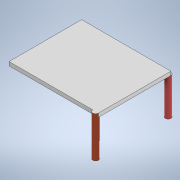
# Autodesk Inventor part: 零件3
Saved by Autodesk Inventor 2022 (Build 260153000, 153)
## iProperties
Created: 2023-03-09
Part Number: 零件3
Material: 一般
Document SubType Name: Modeling
Designer: JOU
Density: 1 g/cm^3
Appearance: 預設
Author: JOU
Autodesk Inventor part; units mm, degrees
ref_plane "YZ Plane" through (0, 0, 0) normal (1, 0, 0) x (0, 1, 0)
ref_plane "XZ Plane" through (0, 0, 0) normal (0, 1, 0) x (-1, 0, 0)
ref_plane "XY Plane" through (0, 0, 0) normal (0, 0, 1) x (1, 0, 0)
sketch "草圖1" plane through (0, 0, 0) normal (0, 1, 0) x (-1, 0, 0)
  circle A0 centre (0.913, -0.7631) radius 0.75
  point P0 (0, 0)
  dimension "d0" = 1.5
  constraints: 1 centre point
  measures "d0" diameter of A0
extrude "擠出1" add sketch "草圖1" along normal blind 10
sketch "草圖2" plane through (-0.913, 10, -0.7631) normal (0, 1, 0) x (1, 0, 0)
  circle A0 centre (0, 0) radius 0.75 projected
  line L0 (-0.75, 0) -> (0.75, 0)
  line L1 (0.75, 0) -> (0.75, 19.5)
  line L2 (0.75, 19.5) -> (-0.75, 19.5)
  line L3 (-0.75, 19.5) -> (-0.75, 0)
  circle A1 centre (0, 0) radius 0.75 projected
  point P0 (0.913, -0.7631)
  dimension "d3" = 19.5
  constraints: 8 end point, 2 parallel, 1 horizontal, 1 horizontal alignment, 1 perpendicular, 1 vertical, 2 other
  measures "d3" distance of L2.end L0.start
extrude "擠出2" add sketch "草圖2" along normal blind 1
pattern_linear "矩形陣列1" count 2 spacing 19.5 along (0, 0, -1) of "擠出1"
sketch "草圖3" plane through (-0.913, 11, -0.7631) normal (0, 1, 0) x (1, 0, 0)
  circle A0 centre (0, 19.5) radius 0.75 projected
  line L0 (-0.75, 19.5) -> (-23.25, 19.5)
  line L1 (-23.25, 19.5) -> (-23.25, 0)
  line L2 (-23.25, 0) -> (-0.75, 0)
  line L3 (-0.75, 0) -> (-0.75, 19.5)
  line L4 (0.75, 0) -> (0.75, 19.5) projected
  point P0 (0.913, -0.7631)
  point P1 (-0.75, 0)
  dimension "d9" = 24
  constraints: 8 end point, 2 parallel, 1 horizontal, 1 perpendicular, 1 point on circle, 1 point on line
  measures "d9" distance between parallel lines of L1 L4
extrude "擠出3" add sketch "草圖3" against normal up to surface (1 mm away) contours L3 L2 L1 L0
